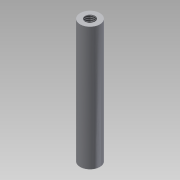
# Autodesk Inventor part: Tube-4mm
Saved by Autodesk Inventor 2014 SP2 (Build 180246200, 246)
## iProperties
Created: 2016-01-22
Part Number: Tube-4mm
Material: Aluminium 6061
Document SubType Name: Modeling
Designer: sd
Density: 2.71 g/cm^3
Appearance: Aluminium - Plat
Mass: 5.10823 g
Surface Area: 19.6035 cm^2
Volume: 1.88496 cm^3
Author: sd
Autodesk Inventor part; units mm, degrees
ref_plane "YZ Plane" through (0, 0, 0) normal (1, 0, 0) x (0, 1, 0)
ref_plane "XZ Plane" through (0, 0, 0) normal (0, 1, 0) x (-1, 0, 0)
ref_plane "XY Plane" through (0, 0, 0) normal (0, 0, 1) x (1, 0, 0)
sketch "Esquisse2" plane through (0, 0, 0) normal (0, 0, 1) x (1, 0, 0)
  circle A0 centre (0, 0) radius 4
  dimension "d4" = 8
  constraints: 1 centre point, 1 coincident
  measures "d4" diameter of A0
extrude "Extrusion2" add sketch "Esquisse2" along normal blind 50
hole "Perçage1" at (0, 0, 50) direction (0, 0, -1) diameter 4 depth 10 tip angle 118
hole "Perçage2" at (0, 0, 0) direction (0, 0, 1) diameter 4 depth 10 tip angle 118
thread "Filetage1" size "M4x0.7" class "6H" standard "ANSI Metric M Profile" full length
thread "Filetage2" size "M4x0.7" class "6H" standard "ANSI Metric M Profile" full length
